Autodesk Inventor part; units mm, degrees
(part 4 of 4)
  line L1533 (32.4501, -1.8935) -> (32.4501, -1.4298) construction
  line L1534 (32.4501, -1.4298) -> (32.4501, -0.1359)
  spline S444 degree 2 poles (32.4501, -0.1359) (32.4501, 0.3044) (33.0931, 0.963) (33.5491, 0.963) knots 0 0 0 1 2 2 2
  line L1535 (32.4501, -0.1359) -> (32.4501, 0.3044) construction
  line L1536 (32.4501, 0.3044) -> (33.0931, 0.963) construction
  line L1537 (33.0931, 0.963) -> (33.5491, 0.963) construction
  line L1538 (33.5491, 0.963) -> (33.8452, 0.963)
  spline S445 degree 2 poles (33.8452, 0.963) (34.2934, 0.963) (34.9442, 0.3239) (34.9442, -0.1359) knots 0 0 0 1 2 2 2
  line L1539 (33.8452, 0.963) -> (34.2934, 0.963) construction
  line L1540 (34.2934, 0.963) -> (34.9442, 0.3239) construction
  line L1541 (34.9442, 0.3239) -> (34.9442, -0.1359) construction
  line L1542 (34.9442, -0.1359) -> (34.9442, -1.4298)
  spline S446 degree 2 poles (34.9442, -1.4298) (34.9442, -1.8779) (34.3051, -2.5288) (33.8452, -2.5288) knots 0 0 0 1 2 2 2
  line L1543 (34.9442, -1.4298) -> (34.9442, -1.8779) construction
  line L1544 (34.9442, -1.8779) -> (34.3051, -2.5288) construction
  line L1545 (34.3051, -2.5288) -> (33.8452, -2.5288) construction
  spline S447 degree 2 poles (36.9396, -2.5288) (36.5381, -2.5288) (35.9419, -1.952) (35.9419, -1.5311) knots 0 0 0 1 2 2 2
  line L1546 (36.9396, -2.5288) -> (36.5381, -2.5288) construction
  line L1547 (36.5381, -2.5288) -> (35.9419, -1.952) construction
  line L1548 (35.9419, -1.952) -> (35.9419, -1.5311) construction
  line L1549 (35.9419, -1.5311) -> (35.9419, -0.0346)
  spline S448 degree 2 poles (35.9419, -0.0346) (35.9419, 0.3785) (36.5265, 0.963) (36.9396, 0.963) knots 0 0 0 1 2 2 2
  line L1550 (35.9419, -0.0346) -> (35.9419, 0.3785) construction
  line L1551 (35.9419, 0.3785) -> (36.5265, 0.963) construction
  line L1552 (36.5265, 0.963) -> (36.9396, 0.963) construction
  line L1553 (36.9396, 0.963) -> (37.6878, 0.963)
  spline S449 degree 2 poles (37.6878, 0.963) (37.7891, 0.963) (37.9372, 0.8111) (37.9372, 0.7136) knots 0 0 0 1 2 2 2
  line L1554 (37.6878, 0.963) -> (37.7891, 0.963) construction
  line L1555 (37.7891, 0.963) -> (37.9372, 0.8111) construction
  line L1556 (37.9372, 0.8111) -> (37.9372, 0.7136) construction
  spline S450 degree 2 poles (37.9372, 0.7136) (37.9372, 0.6279) (37.8125, 0.4642) (37.6878, 0.4642) knots 0 0 0 1 2 2 2
  line L1557 (37.9372, 0.7136) -> (37.9372, 0.6279) construction
  line L1558 (37.9372, 0.6279) -> (37.8125, 0.4642) construction
  line L1559 (37.8125, 0.4642) -> (37.6878, 0.4642) construction
  line L1560 (37.6878, 0.4642) -> (36.9396, 0.4642)
  spline S451 degree 2 poles (36.9396, 0.4642) (36.7291, 0.4642) (36.5849, 0.32) knots 0 0 0 1 1 1
  line L1561 (36.9396, 0.4642) -> (36.7291, 0.4642) construction
  line L1562 (36.7291, 0.4642) -> (36.5849, 0.32) construction
  spline S452 degree 2 poles (36.5849, 0.32) (36.5109, 0.2499) (36.4407, 0.0706) (36.4407, -0.0346) knots 0 0 0 1 2 2 2
  line L1563 (36.5849, 0.32) -> (36.5109, 0.2499) construction
  line L1564 (36.5109, 0.2499) -> (36.4407, 0.0706) construction
  line L1565 (36.4407, 0.0706) -> (36.4407, -0.0346) construction
  line L1566 (36.4407, -0.0346) -> (36.4407, -1.5311)
  spline S453 degree 2 poles (36.4407, -1.5311) (36.4407, -1.7415) (36.5849, -1.8857) knots 0 0 0 1 1 1
  line L1567 (36.4407, -1.5311) -> (36.4407, -1.7415) construction
  line L1568 (36.4407, -1.7415) -> (36.5849, -1.8857) construction
  spline S454 degree 2 poles (36.5849, -1.8857) (36.659, -1.952) (36.7447, -1.9949) knots 0 0 0 1 1 1
  line L1569 (36.5849, -1.8857) -> (36.659, -1.952) construction
  line L1570 (36.659, -1.952) -> (36.7447, -1.9949) construction
  spline S455 degree 2 poles (36.7447, -1.9949) (36.8499, -2.0299) (36.9396, -2.0299) knots 0 0 0 1 1 1
  line L1571 (36.7447, -1.9949) -> (36.8499, -2.0299) construction
  line L1572 (36.8499, -2.0299) -> (36.9396, -2.0299) construction
  line L1573 (36.9396, -2.0299) -> (37.6878, -2.0299)
  spline S456 degree 2 poles (37.6878, -2.0299) (37.7891, -2.0299) (37.9372, -2.1819) (37.9372, -2.2794) knots 0 0 0 1 2 2 2
  line L1574 (37.6878, -2.0299) -> (37.7891, -2.0299) construction
  line L1575 (37.7891, -2.0299) -> (37.9372, -2.1819) construction
  line L1576 (37.9372, -2.1819) -> (37.9372, -2.2794) construction
  spline S457 degree 2 poles (37.9372, -2.2794) (37.9372, -2.3651) (37.8125, -2.5288) (37.6878, -2.5288) knots 0 0 0 1 2 2 2
  line L1577 (37.9372, -2.2794) -> (37.9372, -2.3651) construction
  line L1578 (37.9372, -2.3651) -> (37.8125, -2.5288) construction
  line L1579 (37.8125, -2.5288) -> (37.6878, -2.5288) construction
  line L1580 (37.6878, -2.5288) -> (36.9396, -2.5288)
  circle A18 centre (0, 9) radius 12
  circle A19 centre (0, -73) radius 12
  circle A20 centre (-20, -21) radius 12
  circle A21 centre (31, -45) radius 5.5
  circle A22 centre (20, -21) radius 12
  circle A23 centre (-41, -108) radius 1.5
  circle A24 centre (41, 107) radius 1.5
  circle A25 centre (-41, 107) radius 1.5
  circle A26 centre (41, -108) radius 1.5
  spline S458 degree 2 poles (-23.3397, -51.0373) (-23.1432, -51.2471) (-23.1432, -51.5935) knots 0 0 0 1 1 1
  line L1581 (-23.3397, -51.0373) -> (-23.1432, -51.2471) construction
  line L1582 (-23.1432, -51.2471) -> (-23.1432, -51.5935) construction
  line L1583 (-23.1432, -51.5935) -> (-23.1432, -52.7925)
  spline S459 degree 2 poles (-23.1432, -52.7925) (-23.1432, -53.1222) (-23.6094, -53.5885) (-23.9392, -53.5885) knots 0 0 0 1 2 2 2
  line L1584 (-23.1432, -52.7925) -> (-23.1432, -53.1222) construction
  line L1585 (-23.1432, -53.1222) -> (-23.6094, -53.5885) construction
  line L1586 (-23.6094, -53.5885) -> (-23.9392, -53.5885) construction
  line L1587 (-23.9392, -53.5885) -> (-24.3388, -53.5885)
  spline S460 degree 2 poles (-24.3388, -53.5885) (-24.6652, -53.5885) (-25.1348, -53.1222) (-25.1348, -52.7925) knots 0 0 0 1 2 2 2
  line L1588 (-24.3388, -53.5885) -> (-24.6652, -53.5885) construction
  line L1589 (-24.6652, -53.5885) -> (-25.1348, -53.1222) construction
  line L1590 (-25.1348, -53.1222) -> (-25.1348, -52.7925) construction
  line L1591 (-25.1348, -52.7925) -> (-25.1348, -50.3179)
  spline S461 degree 2 poles (-25.1348, -50.3179) (-25.1348, -49.9815) (-24.9117, -49.7817) knots 0 0 0 1 1 1
  line L1592 (-25.1348, -50.3179) -> (-25.1348, -49.9815) construction
  line L1593 (-25.1348, -49.9815) -> (-24.9117, -49.7817) construction
  spline S462 degree 2 poles (-24.9117, -49.7817) (-24.7085, -49.6018) (-24.4121, -49.6018) knots 0 0 0 1 1 1
  line L1594 (-24.9117, -49.7817) -> (-24.7085, -49.6018) construction
  line L1595 (-24.7085, -49.6018) -> (-24.4121, -49.6018) construction
  spline S463 degree 2 poles (-24.4121, -49.6018) (-24.1223, -49.6018) (-23.9225, -49.7784) knots 0 0 0 1 1 1
  line L1596 (-24.4121, -49.6018) -> (-24.1223, -49.6018) construction
  line L1597 (-24.1223, -49.6018) -> (-23.9225, -49.7784) construction
  spline S464 degree 2 poles (-23.9225, -49.7784) (-23.6994, -49.9782) (-23.6994, -50.3146) knots 0 0 0 1 1 1
  line L1598 (-23.9225, -49.7784) -> (-23.6994, -49.9782) construction
  line L1599 (-23.6994, -49.9782) -> (-23.6994, -50.3146) construction
  spline S465 degree 2 poles (-23.6994, -50.3146) (-23.6994, -50.651) (-23.9392, -50.8108) knots 0 0 0 1 1 1
  line L1600 (-23.6994, -50.3146) -> (-23.6994, -50.651) construction
  line L1601 (-23.6994, -50.651) -> (-23.9392, -50.8108) construction
  spline S466 degree 2 poles (-23.9392, -50.8108) (-23.5528, -50.8108) (-23.3397, -51.0373) knots 0 0 0 1 1 1
  line L1602 (-23.9392, -50.8108) -> (-23.5528, -50.8108) construction
  line L1603 (-23.5528, -50.8108) -> (-23.3397, -51.0373) construction
  line L1604 (-26.8101, -53.5885) -> (-27.0499, -53.5885)
  spline S467 degree 2 poles (-27.0499, -53.5885) (-27.4096, -53.5885) (-27.9258, -53.0756) (-27.9258, -52.7126) knots 0 0 0 1 2 2 2
  line L1605 (-27.0499, -53.5885) -> (-27.4096, -53.5885) construction
  line L1606 (-27.4096, -53.5885) -> (-27.9258, -53.0756) construction
  line L1607 (-27.9258, -53.0756) -> (-27.9258, -52.7126) construction
  line L1608 (-27.9258, -52.7126) -> (-27.9258, -51.6735)
  spline S468 degree 2 poles (-27.9258, -51.6735) (-27.9258, -51.3104) (-27.4096, -50.7975) (-27.0499, -50.7975) knots 0 0 0 1 2 2 2
  line L1609 (-27.9258, -51.6735) -> (-27.9258, -51.3104) construction
  line L1610 (-27.9258, -51.3104) -> (-27.4096, -50.7975) construction
  line L1611 (-27.4096, -50.7975) -> (-27.0499, -50.7975) construction
  line L1612 (-27.0499, -50.7975) -> (-26.8101, -50.7975)
  spline S469 degree 2 poles (-26.8101, -50.7975) (-26.4471, -50.7975) (-25.9342, -51.3104) (-25.9342, -51.6735) knots 0 0 0 1 2 2 2
  line L1613 (-26.8101, -50.7975) -> (-26.4471, -50.7975) construction
  line L1614 (-26.4471, -50.7975) -> (-25.9342, -51.3104) construction
  line L1615 (-25.9342, -51.3104) -> (-25.9342, -51.6735) construction
  line L1616 (-25.9342, -51.6735) -> (-25.9342, -52.7126)
  spline S470 degree 2 poles (-25.9342, -52.7126) (-25.9342, -53.079) (-26.4471, -53.5885) (-26.8101, -53.5885) knots 0 0 0 1 2 2 2
  line L1617 (-25.9342, -52.7126) -> (-25.9342, -53.079) construction
  line L1618 (-25.9342, -53.079) -> (-26.4471, -53.5885) construction
  line L1619 (-26.4471, -53.5885) -> (-26.8101, -53.5885) construction
  spline S471 degree 2 poles (-36.0457, -53.5885) (-36.2889, -53.5885) (-36.572, -53.5452) knots 0 0 0 1 1 1
  line L1620 (-36.0457, -53.5885) -> (-36.2889, -53.5885) construction
  line L1621 (-36.2889, -53.5885) -> (-36.572, -53.5452) construction
  spline S472 degree 2 poles (-36.572, -53.5452) (-36.8051, -53.5086) (-36.9483, -53.3287) knots 0 0 0 1 1 1
  line L1622 (-36.572, -53.5452) -> (-36.8051, -53.5086) construction
  line L1623 (-36.8051, -53.5086) -> (-36.9483, -53.3287) construction
  spline S473 degree 2 poles (-36.9483, -53.3287) (-37.0782, -53.1622) (-37.0782, -52.9457) knots 0 0 0 1 1 1
  line L1624 (-36.9483, -53.3287) -> (-37.0782, -53.1622) construction
  line L1625 (-37.0782, -53.1622) -> (-37.0782, -52.9457) construction
  spline S474 degree 2 poles (-37.0782, -52.9457) (-37.0782, -52.6593) (-36.8584, -52.4728) knots 0 0 0 1 1 1
  line L1626 (-37.0782, -52.9457) -> (-37.0782, -52.6593) construction
  line L1627 (-37.0782, -52.6593) -> (-36.8584, -52.4728) construction
  line L1628 (-36.8584, -52.4728) -> (-35.5861, -51.5969)
  spline S475 degree 2 poles (-35.5861, -51.5969) (-35.5262, -51.5436) (-35.5262, -51.4736) knots 0 0 0 1 1 1
  line L1629 (-35.5861, -51.5969) -> (-35.5262, -51.5436) construction
  line L1630 (-35.5262, -51.5436) -> (-35.5262, -51.4736) construction
  spline S476 degree 2 poles (-35.5262, -51.4736) (-35.5262, -51.3237) (-35.7193, -51.2671) knots 0 0 0 1 1 1
  line L1631 (-35.5262, -51.4736) -> (-35.5262, -51.3237) construction
  line L1632 (-35.5262, -51.3237) -> (-35.7193, -51.2671) construction
  spline S477 degree 2 poles (-35.7193, -51.2671) (-35.9225, -51.2072) (-36.1756, -51.2072) knots 0 0 0 1 1 1
  line L1633 (-35.7193, -51.2671) -> (-35.9225, -51.2072) construction
  line L1634 (-35.9225, -51.2072) -> (-36.1756, -51.2072) construction
  spline S478 degree 2 poles (-36.1756, -51.2072) (-36.5886, -51.2072) (-36.7785, -51.3571) knots 0 0 0 1 1 1
  line L1635 (-36.1756, -51.2072) -> (-36.5886, -51.2072) construction
  line L1636 (-36.5886, -51.2072) -> (-36.7785, -51.3571) construction
  spline S479 degree 2 poles (-36.7785, -51.3571) (-36.8384, -51.4004) (-36.9017, -51.4004) knots 0 0 0 1 1 1
  line L1637 (-36.7785, -51.3571) -> (-36.8384, -51.4004) construction
  line L1638 (-36.8384, -51.4004) -> (-36.9017, -51.4004) construction
  spline S480 degree 2 poles (-36.9017, -51.4004) (-36.9816, -51.4004) (-37.1015, -51.2771) (-37.1015, -51.1939) knots 0 0 0 1 2 2 2
  line L1639 (-36.9017, -51.4004) -> (-36.9816, -51.4004) construction
  line L1640 (-36.9816, -51.4004) -> (-37.1015, -51.2771) construction
  line L1641 (-37.1015, -51.2771) -> (-37.1015, -51.1939) construction
  spline S481 degree 2 poles (-37.1015, -51.1939) (-37.1015, -51.1006) (-37.0183, -51.0373) knots 0 0 0 1 1 1
  line L1642 (-37.1015, -51.1939) -> (-37.1015, -51.1006) construction
  line L1643 (-37.1015, -51.1006) -> (-37.0183, -51.0373) construction
  spline S482 degree 2 poles (-37.0183, -51.0373) (-36.7352, -50.8175) (-36.1423, -50.8175) knots 0 0 0 1 1 1
  line L1644 (-37.0183, -51.0373) -> (-36.7352, -50.8175) construction
  line L1645 (-36.7352, -50.8175) -> (-36.1423, -50.8175) construction
  spline S483 degree 2 poles (-36.1423, -50.8175) (-35.8392, -50.8175) (-35.3796, -50.9541) (-35.1165, -51.2705) (-35.1165, -51.4636) knots 0 0 0 1 2 3 3 3
  line L1646 (-36.1423, -50.8175) -> (-35.8392, -50.8175) construction
  line L1647 (-35.8392, -50.8175) -> (-35.3796, -50.9541) construction
  line L1648 (-35.3796, -50.9541) -> (-35.1165, -51.2705) construction
  line L1649 (-35.1165, -51.2705) -> (-35.1165, -51.4636) construction
  spline S484 degree 2 poles (-35.1165, -51.4636) (-35.1165, -51.7168) (-35.3463, -51.9099) knots 0 0 0 1 1 1
  line L1650 (-35.1165, -51.4636) -> (-35.1165, -51.7168) construction
  line L1651 (-35.1165, -51.7168) -> (-35.3463, -51.9099) construction
  line L1652 (-35.3463, -51.9099) -> (-36.6153, -52.7859)
  spline S485 degree 2 poles (-36.6153, -52.7859) (-36.6885, -52.8458) (-36.6885, -52.9424) knots 0 0 0 1 1 1
  line L1653 (-36.6153, -52.7859) -> (-36.6885, -52.8458) construction
  line L1654 (-36.6885, -52.8458) -> (-36.6885, -52.9424) construction
  spline S486 degree 2 poles (-36.6885, -52.9424) (-36.6885, -53.1256) (-36.512, -53.1522) knots 0 0 0 1 1 1
  line L1655 (-36.6885, -52.9424) -> (-36.6885, -53.1256) construction
  line L1656 (-36.6885, -53.1256) -> (-36.512, -53.1522) construction
  spline S487 degree 2 poles (-36.512, -53.1522) (-36.2622, -53.1922) (-36.0491, -53.1922) knots 0 0 0 1 1 1
  line L1657 (-36.512, -53.1522) -> (-36.2622, -53.1922) construction
  line L1658 (-36.2622, -53.1922) -> (-36.0491, -53.1922) construction
  spline S488 degree 2 poles (-36.0491, -53.1922) (-35.6594, -53.1922) (-35.3996, -53.0523) knots 0 0 0 1 1 1
  line L1659 (-36.0491, -53.1922) -> (-35.6594, -53.1922) construction
  line L1660 (-35.6594, -53.1922) -> (-35.3996, -53.0523) construction
  spline S489 degree 2 poles (-35.3996, -53.0523) (-35.3497, -53.0257) (-35.2997, -53.0257) knots 0 0 0 1 1 1
  line L1661 (-35.3996, -53.0523) -> (-35.3497, -53.0257) construction
  line L1662 (-35.3497, -53.0257) -> (-35.2997, -53.0257) construction
  spline S490 degree 2 poles (-35.2997, -53.0257) (-35.2164, -53.0257) (-35.0999, -53.1522) (-35.0999, -53.2355) knots 0 0 0 1 2 2 2
  line L1663 (-35.2997, -53.0257) -> (-35.2164, -53.0257) construction
  line L1664 (-35.2164, -53.0257) -> (-35.0999, -53.1522) construction
  line L1665 (-35.0999, -53.1522) -> (-35.0999, -53.2355) construction
  spline S491 degree 2 poles (-35.0999, -53.2355) (-35.0999, -53.3487) (-35.2098, -53.4053) knots 0 0 0 1 1 1
  line L1666 (-35.0999, -53.2355) -> (-35.0999, -53.3487) construction
  line L1667 (-35.0999, -53.3487) -> (-35.2098, -53.4053) construction
  spline S492 degree 2 poles (-35.2098, -53.4053) (-35.5528, -53.5885) (-36.0457, -53.5885) knots 0 0 0 1 1 1
  line L1668 (-35.2098, -53.4053) -> (-35.5528, -53.5885) construction
  line L1669 (-35.5528, -53.5885) -> (-36.0457, -53.5885) construction
  line L1670 (-33.1915, -53.5885) -> (-33.4313, -53.5885)
  spline S493 degree 2 poles (-33.4313, -53.5885) (-33.791, -53.5885) (-34.3072, -53.0756) (-34.3072, -52.7126) knots 0 0 0 1 2 2 2
  line L1671 (-33.4313, -53.5885) -> (-33.791, -53.5885) construction
  line L1672 (-33.791, -53.5885) -> (-34.3072, -53.0756) construction
  line L1673 (-34.3072, -53.0756) -> (-34.3072, -52.7126) construction
  line L1674 (-34.3072, -52.7126) -> (-34.3072, -51.6735)
  spline S494 degree 2 poles (-34.3072, -51.6735) (-34.3072, -51.3104) (-33.791, -50.7975) (-33.4313, -50.7975) knots 0 0 0 1 2 2 2
  line L1675 (-34.3072, -51.6735) -> (-34.3072, -51.3104) construction
  line L1676 (-34.3072, -51.3104) -> (-33.791, -50.7975) construction
  line L1677 (-33.791, -50.7975) -> (-33.4313, -50.7975) construction
  line L1678 (-33.4313, -50.7975) -> (-33.1915, -50.7975)
  spline S495 degree 2 poles (-33.1915, -50.7975) (-32.8284, -50.7975) (-32.3155, -51.3104) (-32.3155, -51.6735) knots 0 0 0 1 2 2 2
  line L1679 (-33.1915, -50.7975) -> (-32.8284, -50.7975) construction
  line L1680 (-32.8284, -50.7975) -> (-32.3155, -51.3104) construction
  line L1681 (-32.3155, -51.3104) -> (-32.3155, -51.6735) construction
  line L1682 (-32.3155, -51.6735) -> (-32.3155, -52.7126)
  spline S496 degree 2 poles (-32.3155, -52.7126) (-32.3155, -53.079) (-32.8284, -53.5885) (-33.1915, -53.5885) knots 0 0 0 1 2 2 2
  line L1683 (-32.3155, -52.7126) -> (-32.3155, -53.079) construction
  line L1684 (-32.3155, -53.079) -> (-32.8284, -53.5885) construction
  line L1685 (-32.8284, -53.5885) -> (-33.1915, -53.5885) construction
  spline S497 degree 2 poles (-31.1165, -53.3887) (-31.1165, -53.5885) (-31.3163, -53.5885) knots 0 0 0 1 1 1
  line L1686 (-31.1165, -53.3887) -> (-31.1165, -53.5885) construction
  line L1687 (-31.1165, -53.5885) -> (-31.3163, -53.5885) construction
  spline S498 degree 2 poles (-31.3163, -53.5885) (-31.5162, -53.5885) (-31.5162, -53.3887) knots 0 0 0 1 1 1
  line L1688 (-31.3163, -53.5885) -> (-31.5162, -53.5885) construction
  line L1689 (-31.5162, -53.5885) -> (-31.5162, -53.3887) construction
  line L1690 (-31.5162, -53.3887) -> (-31.5162, -50.9974)
  spline S499 degree 2 poles (-31.5162, -50.9974) (-31.5162, -50.7975) (-31.3163, -50.7975) knots 0 0 0 1 1 1
  line L1691 (-31.5162, -50.9974) -> (-31.5162, -50.7975) construction
  line L1692 (-31.5162, -50.7975) -> (-31.3163, -50.7975) construction
  line L1693 (-31.3163, -50.7975) -> (-29.5212, -50.7975)
  spline S500 degree 2 poles (-29.5212, -50.7975) (-29.1915, -50.7975) (-28.7252, -51.2638) (-28.7252, -51.5935) knots 0 0 0 1 2 2 2
  line L1694 (-29.5212, -50.7975) -> (-29.1915, -50.7975) construction
  line L1695 (-29.1915, -50.7975) -> (-28.7252, -51.2638) construction
  line L1696 (-28.7252, -51.2638) -> (-28.7252, -51.5935) construction
  line L1697 (-28.7252, -51.5935) -> (-28.7252, -53.3887)
  spline S501 degree 2 poles (-28.7252, -53.3887) (-28.7252, -53.5885) (-28.925, -53.5885) knots 0 0 0 1 1 1
  line L1698 (-28.7252, -53.3887) -> (-28.7252, -53.5885) construction
  line L1699 (-28.7252, -53.5885) -> (-28.925, -53.5885) construction
  spline S502 degree 2 poles (-28.925, -53.5885) (-29.1248, -53.5885) (-29.1248, -53.3887) knots 0 0 0 1 1 1
  line L1700 (-28.925, -53.5885) -> (-29.1248, -53.5885) construction
  line L1701 (-29.1248, -53.5885) -> (-29.1248, -53.3887) construction
  line L1702 (-29.1248, -53.3887) -> (-29.1248, -51.5969)
  spline S503 degree 2 poles (-29.1248, -51.5969) (-29.1248, -51.4337) (-29.358, -51.1972) (-29.5212, -51.1972) knots 0 0 0 1 2 2 2
  line L1703 (-29.1248, -51.5969) -> (-29.1248, -51.4337) construction
  line L1704 (-29.1248, -51.4337) -> (-29.358, -51.1972) construction
  line L1705 (-29.358, -51.1972) -> (-29.5212, -51.1972) construction
  spline S504 degree 2 poles (-29.9208, -53.3887) (-29.9208, -53.5885) (-30.1207, -53.5885) knots 0 0 0 1 1 1
  line L1706 (-29.9208, -53.3887) -> (-29.9208, -53.5885) construction
  line L1707 (-29.9208, -53.5885) -> (-30.1207, -53.5885) construction
  spline S505 degree 2 poles (-30.1207, -53.5885) (-30.3205, -53.5885) (-30.3205, -53.3887) knots 0 0 0 1 1 1
  line L1708 (-30.1207, -53.5885) -> (-30.3205, -53.5885) construction
  line L1709 (-30.3205, -53.5885) -> (-30.3205, -53.3887) construction
  arc A27 (-17.2007, 21.4241) -> (-14.617, 23.9079) centre (-16.0265, 22.7884) ccw
  arc A28 (-19.9259, 16.4717) -> (-18.3529, 19.7074) centre (-19.0832, 18.0622) ccw
  arc A29 (-21.0745, 10.9199) -> (-20.3679, 14.4478) centre (-20.7813, 12.6959) ccw
  arc A30 (-21.295, 5.2959) -> (-21.6483, 8.7508) centre (-21, 7.0716) ccw
  line L1710 (-21, 4.2152) -> (-21.0904, 4.5169) construction
  line L1711 (-13.8233, 24.5884) -> (-13.8357, 24.5884) construction
  line L1712 (-21.2894, 10.3973) -> (-21.0971, 10.8642) construction
  line L1713 (-21.0971, 10.8642) -> (-21.0745, 10.9199) construction
  line L1714 (-20.3322, 14.7036) -> (-20.2518, 15.2169) construction
  line L1715 (-20.3679, 14.4478) -> (-20.3322, 14.7036) construction
  spline S506 degree 4 poles (-20.3679, 14.4478) (-20.3322, 14.7036) (-20.2518, 15.2169) (-20.1457, 15.7263) (-20.0047, 16.2255) (-19.9259, 16.4717) knots 4.618445 4.618445 4.618445 4.618445 4.618445 5 5.382136 5.382136 5.382136 5.382136 5.382136
  line L1716 (-20.2518, 15.2169) -> (-20.1457, 15.7263) construction
  line L1717 (-20.1457, 15.7263) -> (-20.0047, 16.2255) construction
  line L1718 (-20.0047, 16.2255) -> (-19.9259, 16.4717) construction
  line L1719 (-18.3179, 19.7661) -> (-18.0708, 20.178) construction
  line L1720 (-18.3529, 19.7074) -> (-18.3179, 19.7661) construction
  spline S507 degree 4 poles (-18.3529, 19.7074) (-18.3179, 19.7661) (-18.0708, 20.178) (-17.8349, 20.5605) (-17.5807, 20.9652) (-17.2007, 21.4241) knots 6.86338 6.86338 6.86338 6.86338 6.86338 7 7.833995 7.833995 7.833995 7.833995 7.833995
  spline S508 degree 4 poles (-14.617, 23.9079) (-14.2914, 24.1893) (-14.0075, 24.4309) (-13.8233, 24.5884) (-13.8357, 24.5884) knots 8.646999 8.646999 8.646999 8.646999 8.646999 9 9 9 9 9
  line L1721 (-18.0708, 20.178) -> (-17.8349, 20.5605) construction
  line L1722 (-17.8349, 20.5605) -> (-17.5807, 20.9652) construction
  line L1723 (-17.5807, 20.9652) -> (-17.2007, 21.4241) construction
  line L1724 (-14.0075, 24.4309) -> (-13.8233, 24.5884) construction
  line L1725 (-14.2914, 24.1893) -> (-14.0075, 24.4309) construction
  line L1726 (-14.617, 23.9079) -> (-14.2914, 24.1893) construction
  spline S509 degree 4 poles (-21, 4.2152) (-21.0904, 4.5169) (-21.1685, 4.7951) (-21.2362, 5.0538) (-21.295, 5.2959) knots 1 1 1 1 1 1.18816 1.18816 1.18816 1.18816 1.18816
  spline S510 degree 4 poles (-21.6483, 8.7508) (-21.606, 9.3484) (-21.4876, 9.9294) (-21.2894, 10.3973) (-21.0971, 10.8642) (-21.0745, 10.9199) knots 2.138213 2.138213 2.138213 2.138213 2.138213 3 3.116481 3.116481 3.116481 3.116481 3.116481
  line L1727 (-21.0904, 4.5169) -> (-21.1685, 4.7951) construction
  line L1728 (-21.1685, 4.7951) -> (-21.2362, 5.0538) construction
  line L1729 (-21.2362, 5.0538) -> (-21.295, 5.2959) construction
  line L1730 (-21.4876, 9.9294) -> (-21.2894, 10.3973) construction
  line L1731 (-21.606, 9.3484) -> (-21.4876, 9.9294) construction
  line L1732 (-21.6483, 8.7508) -> (-21.606, 9.3484) construction
  circle A31 centre (0, 9) radius 13
  line L1733 (-21, 4.2152) -> (-12.0874, 4.2152)
  line L1734 (0, 9) -> (0, 15.2169)
  arc A32 (18.3529, 19.7074) -> (19.9259, 16.4717) centre (19.0832, 18.0622) ccw
  arc A33 (20.3679, 14.4478) -> (21.0745, 10.9199) centre (20.7813, 12.6959) ccw
  arc A34 (21.6483, 8.7508) -> (21.295, 5.2959) centre (21, 7.0716) ccw
  line L1735 (21, 4.2152) -> (21.0904, 4.5169) construction
  line L1736 (21.2894, 10.3973) -> (21.0971, 10.8642) construction
  line L1737 (21.0971, 10.8642) -> (21.0745, 10.9199) construction
  line L1738 (20.3322, 14.7036) -> (20.2518, 15.2169) construction
  line L1739 (20.3679, 14.4478) -> (20.3322, 14.7036) construction
  line L1740 (20.2518, 15.2169) -> (20.1457, 15.7263) construction
  line L1741 (20.1457, 15.7263) -> (20.0047, 16.2255) construction
  line L1742 (20.0047, 16.2255) -> (19.9259, 16.4717) construction
  line L1743 (18.3179, 19.7661) -> (18.0708, 20.178) construction
  line L1744 (18.3529, 19.7074) -> (18.3179, 19.7661) construction
  spline S511 degree 4 poles (20.3679, 14.4478) (20.3322, 14.7036) (20.2518, 15.2169) (20.1457, 15.7263) (20.0047, 16.2255) (19.9259, 16.4717) knots 4.618445 4.618445 4.618445 4.618445 4.618445 5 5.382136 5.382136 5.382136 5.382136 5.382136
  line L1745 (18.0708, 20.178) -> (17.8349, 20.5605) construction
  line L1746 (17.8349, 20.5605) -> (17.5807, 20.9652) construction
  line L1747 (17.5807, 20.9652) -> (17.2007, 21.4241) construction
  spline S512 degree 4 poles (18.3529, 19.7074) (18.3179, 19.7661) (18.0708, 20.178) (17.8349, 20.5605) (17.5807, 20.9652) (17.2007, 21.4241) knots 6.86338 6.86338 6.86338 6.86338 6.86338 7 7.833995 7.833995 7.833995 7.833995 7.833995
  line L1748 (21.0904, 4.5169) -> (21.1685, 4.7951) construction
  line L1749 (21.1685, 4.7951) -> (21.2362, 5.0538) construction
  line L1750 (21.2362, 5.0538) -> (21.295, 5.2959) construction
  line L1751 (21.4876, 9.9294) -> (21.2894, 10.3973) construction
  line L1752 (21.606, 9.3484) -> (21.4876, 9.9294) construction
  line L1753 (21.6483, 8.7508) -> (21.606, 9.3484) construction
  spline S513 degree 4 poles (21, 4.2152) (21.0904, 4.5169) (21.1685, 4.7951) (21.2362, 5.0538) (21.295, 5.2959) knots 1 1 1 1 1 1.18816 1.18816 1.18816 1.18816 1.18816
  spline S514 degree 4 poles (21.6483, 8.7508) (21.606, 9.3484) (21.4876, 9.9294) (21.2894, 10.3973) (21.0971, 10.8642) (21.0745, 10.9199) knots 2.138213 2.138213 2.138213 2.138213 2.138213 3 3.116481 3.116481 3.116481 3.116481 3.116481
  line L1754 (21, 4.2152) -> (12.0874, 4.2152)
  arc A35 (14.617, 23.9079) -> (17.2007, 21.4241) centre (16.0265, 22.7884) ccw
  line L1755 (-13.8233, 24.5884) -> (14.617, 23.9079)
  line L1756 (-13.8357, 24.5884) -> (-13.8233, 24.5884)
  point P0 (0, 0)
  point P1 (-11.6193, 4.2152)
  point P2 (11.6193, 4.2152)
  point P3 (-21, 4.2152)
  dimension "d0" = 3.6
  dimension "d1" = 3.6
  dimension "d2" = 3.6
  dimension "d3" = 3.6
  dimension "d4" = 1
  constraints: 830 end point, 51 point on circle, 36 centre point, 31 symmetric about line, 7 point on line, 3 horizontal, 2 coincident, 1 vertical, 1549 other
  measures "d0" diameter of A27
  measures "d1" diameter of A28
  measures "d2" diameter of A29
  measures "d3" diameter of A30
  measures "d4" radial gap between concentric circles of A31 A18
extrude "Выдавливание1" add sketch "Эскиз1" along normal blind 6 contours L1755 A35 S512 A32 S511 A33 S514 A34 S513 L16 L1754 A31 L1733 L28 S509 A30 S510 A29 S506 A28 S507 A27 S508 L1756
sketch "Эскиз2" plane through (0, 0, 6) normal (0, 0, 1) x (1, 0, 0)
  arc A0 (-17.2007, 21.4241) -> (-14.617, 23.9079) centre (-16.0265, 22.7884) ccw projected
  arc A1 (-19.9259, 16.4717) -> (-18.3529, 19.7074) centre (-19.0832, 18.0622) ccw projected
  arc A2 (-21.0745, 10.9199) -> (-20.3679, 14.4478) centre (-20.7813, 12.6959) ccw projected
  arc A3 (-21.295, 5.2959) -> (-21.6483, 8.7508) centre (-21, 7.0716) ccw projected
  arc A4 (21.6483, 8.7508) -> (21.295, 5.2959) centre (21, 7.0716) ccw projected
  arc A5 (20.3679, 14.4478) -> (21.0745, 10.9199) centre (20.7813, 12.6959) ccw projected
  arc A6 (18.3529, 19.7074) -> (19.9259, 16.4717) centre (19.0832, 18.0622) ccw projected
  arc A7 (14.617, 23.9079) -> (17.2007, 21.4241) centre (16.0265, 22.7884) ccw projected
  circle A8 centre (-20.7813, 12.6959) radius 1.8
  arc A9 (-21.295, 5.2959) -> (-21.6483, 8.7508) centre (-21, 7.0716) ccw projected
  circle A10 centre (-21, 7.0716) radius 1.8
  circle A11 centre (-19.0832, 18.0622) radius 1.8
  circle A12 centre (-16.0265, 22.7884) radius 1.8
  circle A13 centre (16.0265, 22.7884) radius 1.8
  circle A14 centre (19.0832, 18.0622) radius 1.8
  circle A15 centre (20.7813, 12.6959) radius 1.8
  circle A16 centre (21, 7.0716) radius 1.8
  arc A17 (12.0874, 4.2152) -> (-12.0874, 4.2152) centre (0, 9) ccw projected
  line L0 (-17.6841, 26.3102) -> (17.6841, 26.3102)
  line L1 (-24.2791, 4.2152) -> (24.2791, 4.2152)
  arc A18 (-17.6841, 26.3102) -> (-24.2791, 4.2152) centre (0, 9) ccw
  arc A19 (24.2791, 4.2152) -> (17.6841, 26.3102) centre (0, 9) ccw
  point P0 (0, 0)
  point P1 (-12.0874, 4.2152)
  point P2 (12.0874, 4.2152)
  point P3 (21.0745, 10.9199)
  point P4 (17.2007, 21.4241)
  point P5 (-20.3679, 14.4478)
  point P6 (19.9259, 16.4717)
  point P7 (21.295, 5.2959)
  constraints: 9 coincident, 6 centre point, 4 end point, 4 point on circle, 3 concentric, 2 horizontal, 12 other
extrude "Выдавливание2" add sketch "Эскиз2" along normal blind 2 contours A17 L1 A18 L0 A19
